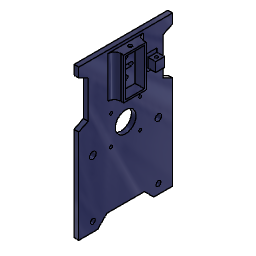
Carro_Y_V4 v6 (Autodesk Fusion 360 design; units mm, degrees)
Autodesk Fusion 360 part; units mm, degrees
note: some values were not read from the file. Set by a fixed rule: which sketch regions a step uses.
sketch "carro eje" plane through (0, 0, 0) normal (1, 0, 0) x (0, 1, 0)
  line L0 (100, 100) -> (100, 0)
  line L1 (100, 0) -> (80, 0)
  line L2 (80, 0) -> (70, 10)
  line L3 (70, 10) -> (30, 10)
  line L4 (30, 10) -> (20, 0)
  line L5 (20, 0) -> (0, 0)
  line L6 (0, 0) -> (0, 100)
  line L7 (15, 71) -> (85, 71) construction
  line L8 (85, 71) -> (85, 10) construction
  line L9 (85, 10) -> (15, 10) construction
  line L10 (15, 10) -> (15, 71) construction
  circle A0 centre (15, 71) radius 3.5
  circle A1 centre (85, 71) radius 3.5
  circle A2 centre (15, 10) radius 2.55
  circle A3 centre (85, 10) radius 2.55
  line L11 (34.5, 100) -> (65.5, 100) construction
  line L12 (65.5, 100) -> (65.5, 69) construction
  line L13 (65.5, 69) -> (34.5, 69) construction
  line L14 (34.5, 69) -> (34.5, 100) construction
  circle A4 centre (34.5, 100) radius 1.55
  circle A5 centre (65.5, 100) radius 1.55
  circle A6 centre (65.5, 69) radius 1.55
  circle A7 centre (34.5, 69) radius 1.55
  line L15 (0, 100) -> (10, 105)
  line L16 (10, 105) -> (10, 145)
  line L17 (10, 145) -> (0, 150)
  line L18 (0, 150) -> (0, 160)
  line L19 (0, 160) -> (100, 160)
  line L20 (100, 160) -> (100, 150)
  line L21 (100, 150) -> (90, 145)
  line L22 (90, 145) -> (90, 105)
  line L23 (90, 105) -> (100, 100)
  circle A8 centre (50, 84.5) radius 11.05
  line L24 (34.5, 100) -> (65.5, 69) construction
  line L25 (50, 145) -> (50, 125) construction
  line L26 (10, 145) -> (90, 145) construction
  circle A9 centre (50, 145) radius 2.55
  circle A10 centre (50, 125) radius 2.55
  line L27 (40, 135) -> (60, 135) construction
  dimension "d4" = 100
  dimension "d5" = 20
  dimension "d6" = 40
  dimension "d7" = 10
  dimension "d8" = 100
  dimension "d11" = 61
  dimension "d12" = 70
  dimension "d13" = 15
  dimension "d14" = 10
  dimension "d15" = 5.1
  dimension "d16" = 5.1
  dimension "d17" = 7
  dimension "d18" = 7
  dimension "d19" = 31
  dimension "d20" = 3.1
  dimension "d27" = 10
  dimension "d36" = 40
  dimension "d37" = 40
  dimension "d38" = 100
  dimension "d39" = 10
  dimension "d41" = 160
  dimension "d43" = 10
  dimension "d44" = 60
  dimension "d45" = 22.1
  dimension "d46" = 50
  dimension "d48" = 20
  dimension "d49" = 5.1
  dimension "d50" = 20
  dimension "d52" = 10
  dimension "d53" = 10
  constraint perpendicular L0 L1
  constraint coincident L5.end L6.start
  constraint parallel L3 L5
  constraint perpendicular L5 L6
  constraint equal L1 L5
  constraint equal L0 L6
  constraint equal L2 L4
  constraint horizontal L7
  constraint vertical L8
  constraint horizontal L9
  constraint vertical L10
  constraint coincident L7.start L10.end
  constraint coincident L7.end L8.start
  constraint coincident L9.end L10.start
  constraint coincident L8.end L9.start
  constraint horizontal L11
  constraint vertical L12
  constraint horizontal L13
  constraint vertical L14
  constraint equal L11 L14
  constraint coincident L11.start L14.end
  constraint coincident L11.end L12.start
  constraint coincident L12.end L13.start
  constraint coincident L13.end L14.start
  constraint equal A4 A5
  constraint equal A5 A7
  constraint equal A6 A7
  constraint parallel L6 L16
  constraint parallel L16 L18
  constraint perpendicular L18 L19
  constraint perpendicular L19 L20
  constraint equal L18 L20
  constraint horizontal L19
  constraint equal L15 L17
  constraint equal L15 L23
  constraint equal L21 L23
  constraint vertical L22
  constraint coincident A8.centre L24
  constraint midpoint A8.centre L24
  constraint perpendicular L19 L25
  constraint midpoint L25.start L26
  constraint coincident L25.start A9.centre
  constraint coincident L25.end A10.centre
  constraint equal A9 A10
  constraint perpendicular L25 L27
  measures "d4" distance of L5.end L0.end
  measures "d5" distance of L4.end L5.end
  measures "d6" distance of L2.end L3.end
  measures "d7" vertical distance of L1.end L2.end
  measures "d8" distance of L5.end L6.end
  measures "d11" distance of L7 L9
  measures "d12" distance of L7.start L7.end
  measures "d13" horizontal distance of L0.end L8.end
  measures "d14" vertical distance of L0.end L8.end
  measures "d15" diameter of A2
  measures "d16" diameter of A3
  measures "d17" diameter of A0
  measures "d18" diameter of A1
  measures "d19" distance of L11.start L11.end
  measures "d20" diameter of A4
  measures "d27" horizontal distance of L1.end L2.end
  measures "d36" distance of L15.end L16.end
  measures "d37" distance of L21.end L22.end
  measures "d38" distance of L18.end L19.end
  measures "d39" distance of L17.end L18.end
  measures "d41" vertical distance of L5.end L18.end
  measures "d43" horizontal distance of L20.end L21.end
  measures "d44" vertical distance of L11.end L19.end
  measures "d45" diameter of A8
  measures "d46" horizontal distance of L0.start A8.centre
  measures "d48" distance of L25.start L25.end
  measures "d49" diameter of A9
  measures "d50" distance of L27.start L27.end
  measures "d52" horizontal distance of L25.start L27.end
  measures "d53" vertical distance of L25.end L27.end
extrude "Extrude1" add sketch "carro eje" along normal blind 5
sketch "Sketch9" plane through (5, 0, 0) normal (1, 0, 0) x (0, 1, 0)
  circle A0 centre (85, 71) radius 3.5
  circle A1 centre (15, 71) radius 3.5
  circle A2 centre (34.5, 100) radius 1.55
  circle A3 centre (85, 10) radius 2.55
  circle A4 centre (15, 10) radius 2.55
  circle A5 centre (65.5, 69) radius 1.55
  circle A6 centre (34.5, 69) radius 1.55
  circle A7 centre (65.5, 100) radius 1.55
  circle A8 centre (50, 145) radius 2.55
  circle A9 centre (50, 125) radius 2.55
  circle A10 centre (50, 84.5) radius 11.05
  line L0 (90, 105) -> (90, 145)
  line L1 (90, 145) -> (100, 150)
  line L2 (100, 150) -> (100, 160)
  line L3 (100, 160) -> (0, 160)
  line L4 (0, 160) -> (0, 150)
  line L5 (0, 150) -> (10, 145)
  line L6 (10, 145) -> (10, 105)
  line L7 (10, 105) -> (0, 100)
  line L8 (0, 100) -> (0, 0)
  line L9 (0, 0) -> (20, 0)
  line L10 (20, 0) -> (30, 10)
  line L11 (30, 10) -> (70, 10)
  line L12 (70, 10) -> (80, 0)
  line L13 (80, 0) -> (100, 0)
  line L14 (100, 0) -> (100, 100)
  line L15 (100, 100) -> (90, 105)
  line L16 (72, 134) -> (81.5, 134)
  line L17 (81.5, 134) -> (81.5, 124)
  line L18 (81.5, 124) -> (72, 124)
  line L19 (72, 124) -> (72, 134)
  dimension "d122" = 10
  dimension "d123" = 9.5
  dimension "d124" = 8.5
  dimension "d125" = 11
  constraint horizontal L16
  constraint vertical L17
  constraint horizontal L18
  constraint vertical L19
  measures "d122" distance of L16.start L18.end
  measures "d123" distance of L16.start L16.end
  measures "d124" horizontal distance of L0.end L16.end
  measures "d125" vertical distance of L0.end L16.end
extrude "Extrude5" add sketch "Sketch9" along normal blind 10 contours L16 L17 L18 L19
sketch "Sketch10" plane through (5, 0, 0) normal (1, 0, 0) x (0, 1, 0)
  line L0 (72, 124) -> (72, 134)
  line L1 (72, 134) -> (81.5, 134)
  line L2 (81.5, 134) -> (81.5, 124)
  line L3 (81.5, 124) -> (72, 124)
  circle A0 centre (85, 71) radius 3.5
  circle A1 centre (15, 71) radius 3.5
  circle A2 centre (34.5, 100) radius 1.55
  circle A3 centre (85, 10) radius 2.55
  circle A4 centre (15, 10) radius 2.55
  circle A5 centre (65.5, 69) radius 1.55
  circle A6 centre (34.5, 69) radius 1.55
  circle A7 centre (65.5, 100) radius 1.55
  circle A8 centre (50, 145) radius 2.55
  circle A9 centre (50, 125) radius 2.55
  circle A10 centre (50, 84.5) radius 11.05
  line L4 (90, 105) -> (90, 145)
  line L5 (90, 145) -> (100, 150)
  line L6 (100, 150) -> (100, 160)
  line L7 (100, 160) -> (0, 160)
  line L8 (0, 160) -> (0, 150)
  line L9 (0, 150) -> (10, 145)
  line L10 (10, 145) -> (10, 105)
  line L11 (10, 105) -> (0, 100)
  line L12 (0, 100) -> (0, 0)
  line L13 (0, 0) -> (20, 0)
  line L14 (20, 0) -> (30, 10)
  line L15 (30, 10) -> (70, 10)
  line L16 (70, 10) -> (80, 0)
  line L17 (80, 0) -> (100, 0)
  line L18 (100, 0) -> (100, 100)
  line L19 (100, 100) -> (90, 105)
  line L20 (72, 124) -> (81.5, 124)
  line L21 (81.5, 124) -> (81.5, 121)
  line L22 (79.5, 119) -> (74, 119)
  line L23 (72, 121) -> (72, 124)
  arc A11 (72, 121) -> (74, 119) centre (74, 121) ccw
  arc A12 (79.5, 119) -> (81.5, 121) centre (79.5, 121) ccw
  dimension "d128" = 2
  constraint horizontal L20
  constraint vertical L21
  constraint horizontal L22
  constraint vertical L23
  constraint coincident L0.start L3.end
  constraint coincident L2.end L3.start
  constraint tangent L22 A11
  constraint tangent L23 A11
  constraint tangent L22 A12
  constraint tangent L21 A12
  constraint equal A11 A12
  measures "d128" radius of A11
extrude "Extrude6" cut sketch "Sketch10" against normal blind 15 contours L3 L20 L21 L22 L23 A11 A12
fillet "Fillet1" radius 2 3 edges at (5, 81.5, 129) (5, 76.75, 134) (5, 72, 129)
sketch "Sketch11" plane through (0, 0, 134) normal (0, 0, 1) x (-1, 0, 0)
  line L0 (-7, -81.5) -> (-7, -72)
  line L1 (-7, -72) -> (-15, -72)
  line L2 (-15, -72) -> (-15, -81.5)
  line L3 (-15, -81.5) -> (-7, -81.5)
  circle A0 centre (-11, -76.7886) radius 1.55
  dimension "d132" = 3.1
  measures "d132" diameter of A0
extrude "Extrude7" cut sketch "Sketch11" against normal blind 14 contours A0
sketch "Sketch12" plane through (5, 0, 0) normal (1, 0, 0) x (0, 1, 0)
  line L0 (90, 105) -> (90, 145)
  line L1 (90, 145) -> (100, 150)
  line L2 (100, 150) -> (100, 160)
  line L3 (100, 160) -> (0, 160)
  line L4 (0, 160) -> (0, 150)
  line L5 (0, 150) -> (10, 145)
  line L6 (10, 145) -> (10, 105)
  line L7 (10, 105) -> (0, 100)
  line L8 (0, 100) -> (0, 0)
  line L9 (0, 0) -> (20, 0)
  line L10 (20, 0) -> (30, 10)
  line L11 (30, 10) -> (70, 10)
  line L12 (70, 10) -> (80, 0)
  line L13 (80, 0) -> (100, 0)
  line L14 (100, 0) -> (100, 100)
  line L15 (100, 100) -> (90, 105)
  circle A0 centre (50, 84.5) radius 11.05
  circle A1 centre (50, 125) radius 2.55
  circle A2 centre (50, 145) radius 2.55
  circle A3 centre (65.5, 100) radius 1.55
  circle A4 centre (34.5, 69) radius 1.55
  circle A5 centre (65.5, 69) radius 1.55
  circle A6 centre (15, 10) radius 2.55
  circle A7 centre (85, 10) radius 2.55
  circle A8 centre (34.5, 100) radius 1.55
  circle A9 centre (15, 71) radius 3.5
  circle A10 centre (85, 71) radius 3.5
  line L16 (72, 124) -> (70, 124)
  line L17 (70, 124) -> (70, 136)
  line L18 (70, 136) -> (83.5, 136)
  line L19 (83.5, 136) -> (83.5, 124)
  line L20 (83.5, 124) -> (81.5, 124)
  line L21 (81.5, 124) -> (81.5, 121)
  arc A11 (79.5, 119) -> (81.5, 121) centre (79.5, 121) ccw
  line L22 (79.5, 119) -> (74, 119)
  arc A12 (72, 121) -> (74, 119) centre (74, 121) ccw
  line L23 (72, 121) -> (72, 124)
  line L24 (40, 155) -> (60, 155)
  line L25 (60, 155) -> (60, 115)
  line L26 (60, 115) -> (40, 115)
  line L27 (40, 115) -> (40, 155)
  line L28 (38, 157) -> (62, 157)
  line L29 (62, 157) -> (62, 113)
  line L30 (62, 113) -> (38, 113)
  line L31 (38, 113) -> (38, 157)
  dimension "d135" = 20
  dimension "d136" = 40
  dimension "d137" = 10
  dimension "d138" = 10
  dimension "d139" = 24
  dimension "d140" = 44
  dimension "d141" = 2
  dimension "d142" = 2
  constraint horizontal L24
  constraint vertical L25
  constraint horizontal L26
  constraint vertical L27
  constraint horizontal L28
  constraint vertical L29
  constraint horizontal L30
  constraint vertical L31
  measures "d135" distance of L24.start L24.end
  measures "d136" distance of L24.start L26.end
  measures "d137" vertical distance of A2.centre L24.end
  measures "d138" horizontal distance of A2.centre L24.end
  measures "d139" distance of L28.start L28.end
  measures "d140" distance of L28.end L29.end
  measures "d141" vertical distance of L25.end L29.end
  measures "d142" horizontal distance of L25.end L29.end
extrude "Extrude8" add sketch "Sketch12" along normal blind 10 contours L28 L29 L30 L31
fillet "Fillet2" radius 7 2 edges at (5, 38, 135) (5, 62, 135)
sketch "Sketch13" plane through (5, 0, 0) normal (1, 0, 0) x (0, 1, 0)
  line L0 (60, 115) -> (60, 155)
  line L1 (60, 155) -> (40, 155)
  line L2 (40, 155) -> (40, 115)
  line L3 (40, 115) -> (60, 115)
  circle A0 centre (50, 125) radius 2.55
  circle A1 centre (50, 145) radius 2.55
  line L4 (46.6, 152.5) -> (53.6, 152.5)
  line L5 (53.6, 152.5) -> (53.6, 150.5)
  line L6 (53.6, 150.5) -> (46.6, 150.5)
  line L7 (46.6, 150.5) -> (46.6, 152.5)
  line L8 (44, 133) -> (56, 133)
  arc A2 (56, 133) -> (56, 137) centre (56, 135) ccw
  line L9 (56, 137) -> (44, 137)
  arc A3 (44, 137) -> (44, 133) centre (44, 135) ccw
  line L10 (44, 135) -> (56, 135) construction
  dimension "d146" = 7
  dimension "d147" = 2
  dimension "d148" = 6.6
  dimension "d149" = 2.5
  dimension "d150" = 10
  dimension "d151" = 12
  dimension "d152" = 6
  constraint horizontal L4
  constraint vertical L5
  constraint horizontal L6
  constraint vertical L7
  constraint tangent L8 A2
  constraint tangent A2 L9
  constraint parallel L8 L9
  constraint tangent L9 A3
  constraint tangent L8 A3
  constraint perpendicular L2 L10
  measures "d146" distance of L4.start L4.end
  measures "d147" distance of L4.start L6.end
  measures "d148" horizontal distance of L1.end L4.start
  measures "d149" vertical distance of L1.end L4.start
  measures "d150" vertical distance of A0.centre A3.centre
  measures "d151" distance of A3.centre A2.centre
  measures "d152" horizontal distance of A0.centre A2.centre
extrude "Extrude9" cut sketch "Sketch13" against normal blind 10 contours L4 L5 L6 L7 | L8 A2 L9 A3
sketch "Sketch14" plane through (0, 0, 157) normal (0, 0, 1) x (-1, 0, 0)
  line L0 (-5, -69) -> (-5, -31)
  arc A0 (-12, -38) -> (-5, -31) centre (-12, -31) ccw
  line L1 (-12, -38) -> (-15, -38)
  line L2 (-15, -38) -> (-15, -62)
  line L3 (-15, -62) -> (-12, -62)
  arc A1 (-5, -69) -> (-12, -62) centre (-12, -69) ccw
  circle A2 centre (-10, -50) radius 2
  dimension "d155" = 4
  measures "d155" diameter of A2
extrude "Extrude10" cut sketch "Sketch14" against normal blind 4 contours A2
fillet "Fillet3" radius 1.5 4 edges at (5, 50.1, 152.5) (5, 46.6, 151.5) (5, 50.1, 150.5) (5, 53.6, 151.5)
sketch "rueda POM" plane through (0, 0, 0) normal (0, 1, 0) x (1, 0, 0)
  line L0 (-2.445, -11.94) -> (3.445, -11.94)
  line L1 (3.445, -11.94) -> (5.615, -9.77)
  line L2 (5.615, -9.77) -> (5.615, -7.94)
  line L3 (5.615, -7.94) -> (1, -7.94)
  line L4 (1, -7.94) -> (1, 0)
  line L5 (1, 0) -> (0, 0)
  line L6 (0, 0) -> (0, -7.94)
  line L7 (0, -7.94) -> (-4.615, -7.94)
  line L8 (-4.615, -7.94) -> (-4.615, -9.77)
  line L9 (-4.615, -9.77) -> (-2.445, -11.94)
  dimension "d59" = 10.23
  dimension "d60" = 135
  dimension "d61" = 135
  dimension "d68" = 5.89
  dimension "d69" = 1
  dimension "d73" = 4
  dimension "d75" = 9.77
  constraint horizontal L0
  constraint perpendicular L0 L2
  constraint perpendicular L2 L3
  constraint perpendicular L3 L4
  constraint perpendicular L4 L5
  constraint perpendicular L5 L6
  constraint perpendicular L4 L7
  constraint equal L1 L9
  constraint equal L2 L8
  constraint equal L3 L7
  constraint equal L4 L6
  constraint coincident L5.end L6.start
  measures "d59" horizontal distance of L1.end L8.end
  measures "d60" angle of L8 L9
  measures "d61" angle of L1 L2
  measures "d68" distance of L0.start L0.end
  measures "d69" distance of L4.end L5.end
  measures "d73" vertical distance of L0.start L7.end
  measures "d75" vertical distance of L1.end L4.end
revolve "Revolve3" [suppressed]
other "CylinderPrimitive1"
sketch "Sketch4" plane through (0, 0, 0) normal (1, 0, 0) x (0, 1, 0)
  line L0 (0, 5.7735) -> (-5, 2.8868)
  line L1 (-5, 2.8868) -> (-5, -2.8868)
  line L2 (-5, -2.8868) -> (0, -5.7735)
  line L3 (0, -5.7735) -> (5, -2.8868)
  line L4 (5, -2.8868) -> (5, 2.8868)
  line L5 (5, 2.8868) -> (0, 5.7735)
  dimension "d79" = 10
  constraint vertical L4
  measures "d79" distance of L0.end L4.end
extrude "Extrude2" [suppressed]
sketch "Sketch5" plane through (6.35, 0, 0) normal (1, 0, 0) x (0, 1, 0)
  line L0 (5, 2.8868) -> (0, 5.7735)
  line L1 (0, 5.7735) -> (-5, 2.8868)
  line L2 (-5, 2.8868) -> (-5, -2.8868)
  line L3 (-5, -2.8868) -> (0, -5.7735)
  line L4 (0, -5.7735) -> (5, -2.8868)
  line L5 (5, -2.8868) -> (5, 2.8868)
  circle A0 centre (0, 0) radius 3.555
  dimension "d83" = 7.11
  constraint coincident A0.centre origin
  measures "d83" diameter of A0
extrude "Extrude3" [suppressed]
sketch "Sketch6" plane through (8.85, 0, 0) normal (1, 0, 0) x (0, 1, 0)
  circle A0 centre (0, 0) radius 3.555
  circle A1 centre (0.79, 0) radius 2.55
  dimension "d86" = 5.1
  dimension "d87" = 0.79
  measures "d86" diameter of A1
  measures "d87" distance of A0.centre A1.centre
extrude "Extrude4" [suppressed]
chamfer "Chamfer1" [suppressed]
chamfer "Chamfer2" [suppressed]
other "BoxPrimitive1"
copy_body "Body->Comp1" [suppressed] in component "carro eje"
copy_body "Body->Comp2" [suppressed] in component "Tuerca excentrica"
named bodies: "carro eje Y Izquierda", "rueda V-slot", "Tuerca excentrica", "carro eje"
